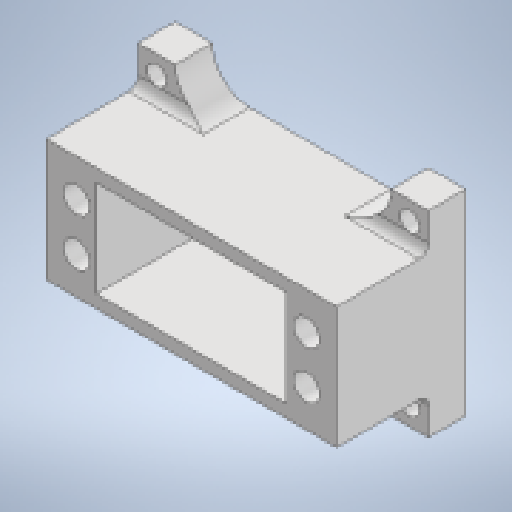
# Autodesk Inventor part: Soporte_Servo
Saved by Autodesk Inventor 2024 (Build 280153000, 153)
## iProperties
Created: 2024-07-18
Part Number: Soporte_Servo
Material: Genérico
Document SubType Name: Modelado
Designer: sergi
Density: 1 g/cm^3
Appearance: Valor por defecto
Sheet Metal Rule: Por defecto
Author: sergi
Autodesk Inventor part; units mm, degrees
ref_plane "YZ Plane" through (0, 0, 0) normal (1, 0, 0) x (0, 1, 0)
ref_plane "XZ Plane" through (0, 0, 0) normal (0, 1, 0) x (-1, 0, 0)
sketch "Boceto1" plane through (0, 0, 0) normal (0, 0, 1) x (1, 0, 0)
  line L0 (-20.0665, -74.268) -> (20.3335, -74.268) projected
  line L1 (-20.0665, -54.068) -> (-20.0665, -74.268) projected
  line L2 (20.3335, -74.268) -> (20.3335, -54.068) projected
  circle A0 centre (24.7835, -69.268) radius 2.2 projected
  circle A1 centre (24.7835, -59.068) radius 2.2 projected
  line L3 (20.3335, -54.068) -> (20.3335, -74.268) projected
  line L4 (20.3335, -54.068) -> (28.3335, -54.068) projected
  line L5 (28.3335, -54.068) -> (28.3335, -74.268) projected
  line L6 (20.3335, -74.268) -> (28.3335, -74.268) projected
  line L7 (-20.0665, -74.268) -> (-28.0665, -74.268) projected
  circle A2 centre (-24.5165, -69.268) radius 2.2 projected
  circle A3 centre (-24.5165, -59.068) radius 2.2 projected
  line L8 (-20.0665, -54.068) -> (-20.0665, -74.268) projected
  line L9 (-20.0665, -54.068) -> (-28.0665, -54.068) projected
  line L10 (-28.0665, -74.268) -> (-28.0665, -54.068) projected
  line L11 (-20.0665, -74.268) -> (-28.0665, -74.268) projected
  line L12 (-20.0665, -66.768) -> (-25.0665, -66.768) projected
  line L13 (-25.0665, -61.568) -> (-25.0665, -66.768) projected
  line L14 (-20.0665, -61.568) -> (-25.0665, -61.568) projected
  line L15 (-20.0665, -54.068) -> (-20.0665, -74.268) projected
  line L16 (20.3335, -54.068) -> (-20.0665, -54.068) projected
  line L17 (20.3335, -74.268) -> (20.3335, -54.068) projected
  line L18 (-20.0665, -74.268) -> (20.3335, -74.268) projected
  circle A4 centre (-10.3665, -64.168) radius 3.1 projected
  line L19 (-28.0665, -74.268) -> (-28.0665, -77.268)
  line L20 (-28.0665, -77.268) -> (-31.0665, -77.268)
  line L21 (28.3335, -54.068) -> (31.3335, -54.068)
  line L22 (31.3335, -54.068) -> (31.3335, -51.068)
  line L23 (31.3335, -51.068) -> (28.3335, -51.068)
  line L24 (28.3335, -51.068) -> (28.3335, -54.068)
  line L25 (31.3335, -51.068) -> (-31.0665, -51.068)
  line L26 (-31.0665, -51.068) -> (-31.0665, -77.268)
  line L27 (-31.0665, -77.268) -> (31.3335, -77.268)
  line L28 (31.3335, -77.268) -> (31.3335, -51.068)
  line L29 (-31.0665, -51.068) -> (-23.0665, -51.068)
  line L30 (-23.0665, -51.068) -> (-23.0665, -43.068)
  line L31 (-23.0665, -43.068) -> (-31.0665, -43.068)
  line L32 (-31.0665, -43.068) -> (-31.0665, -51.068)
  line L33 (-31.0665, -77.268) -> (-23.0665, -77.268)
  line L34 (-23.0665, -77.268) -> (-23.0665, -85.268)
  line L35 (-23.0665, -85.268) -> (-31.0665, -85.268)
  line L36 (-31.0665, -85.268) -> (-31.0665, -77.268)
  line L37 (31.3335, -77.268) -> (23.3335, -77.268)
  line L38 (23.3335, -77.268) -> (23.3335, -85.268)
  line L39 (23.3335, -85.268) -> (31.3335, -85.268)
  line L40 (31.3335, -85.268) -> (31.3335, -77.268)
  line L41 (31.3335, -51.068) -> (23.3335, -51.068)
  line L42 (23.3335, -51.068) -> (23.3335, -43.068)
  line L43 (23.3335, -43.068) -> (31.3335, -43.068)
  line L44 (31.3335, -43.068) -> (31.3335, -51.068)
  line L45 (-27.0665, -43.068) -> (-27.0665, -47.068)
  circle A5 centre (-27.0665, -47.068) radius 2.1
  line L46 (-27.0665, -85.268) -> (-27.0665, -81.268)
  circle A6 centre (-27.0665, -81.268) radius 2.1
  line L47 (27.3335, -43.068) -> (27.3335, -47.068)
  circle A7 centre (27.3335, -47.068) radius 2.1
  line L48 (27.3335, -85.268) -> (27.3335, -81.268)
  circle A8 centre (27.3335, -81.268) radius 2.1
  line L49 (-28.0665, -54.068) -> (28.3335, -54.068)
  line L50 (28.3335, -54.068) -> (28.3335, -74.268)
  line L51 (28.3335, -74.268) -> (-28.0665, -74.268)
  line L52 (-28.0665, -74.268) -> (-28.0665, -54.068)
  line L53 (28.5835, -53.818) -> (-28.3165, -53.818)
  line L54 (-28.3165, -53.818) -> (-28.3165, -74.518)
  line L55 (-28.3165, -74.518) -> (28.5835, -74.518)
  line L56 (28.5835, -74.518) -> (28.5835, -53.818)
  line L57 (-20.3165, -53.818) -> (-20.3165, -74.518)
  line L58 (20.5835, -74.518) -> (20.5835, -53.818)
  line L59 (-25.0665, -61.568) -> (-20.0665, -66.768)
  line L60 (-19.0665, -69.168) -> (-26.0665, -69.168)
  line L61 (-26.0665, -69.168) -> (-26.0665, -59.168)
  line L62 (-26.0665, -59.168) -> (-19.0665, -59.168)
  line L63 (-19.0665, -59.168) -> (-19.0665, -69.168)
  line L64 (-19.0665, -69.168) -> (-26.0665, -59.168) construction
  line L65 (-26.0665, -69.168) -> (-19.0665, -59.168) construction
  point P0 (0, 0)
  point P1 (28.5835, -54.068)
  point P2 (28.3335, -53.818)
  point P3 (-20.3165, -61.568)
  point P4 (-20.3165, -66.768)
  point P5 (-22.5665, -64.168)
  point P6 (-20.3165, -69.168)
  point P7 (-20.3165, -59.168)
  dimension "d0" = 3
  dimension "d1" = 3
  dimension "d2" = 3
  dimension "d3" = 3
  dimension "d4" = 8
  dimension "d5" = 8
  dimension "d6" = 8
  dimension "d7" = 8
  dimension "d8" = 8
  dimension "d9" = 8
  dimension "d10" = 8
  dimension "d11" = 8
  dimension "d12" = 4
  dimension "d13" = 4.2
  dimension "d14" = 4
  dimension "d15" = 4.2
  dimension "d16" = 4
  dimension "d17" = 4.2
  dimension "d18" = 4
  dimension "d19" = 4.2
  dimension "d20" = 0.25
  dimension "d28" = 0.25
  dimension "d29" = 0.25
  dimension "d30" = 7
  dimension "d31" = 10
  constraints: 94 end point, 20 parallel, 10 perpendicular, 8 horizontal, 5 midpoint, 5 vertical, 4 centre point, 4 coincident, 4 point on line, 3 other
  measures "d0" distance of L7.end L19.end
  measures "d1" distance of L19.end L20.end
  measures "d2" distance of L23.end L22.end
  measures "d3" distance of L22.end L21.end
  measures "d4" distance of L31.end L30.end
  measures "d5" distance of L30.end L29.end
  measures "d6" distance of L34.end L35.end
  measures "d7" distance of L33.end L34.end
  measures "d8" distance of L39.end L38.end
  measures "d9" distance of L38.end L37.end
  measures "d10" distance of L42.end L43.end
  measures "d11" distance of L41.end L42.end
  measures "d12" distance of L45.start L45.end
  measures "d13" diameter of A5
  measures "d14" distance of L46.start L46.end
  measures "d15" diameter of A6
  measures "d16" distance of L47.start L47.end
  measures "d17" diameter of A7
  measures "d18" distance of L48.start L48.end
  measures "d19" diameter of A8
  measures "d20" distance between parallel lines of L49 L53
  measures "d28" distance between parallel lines of L1 L57
  measures "d29" distance between parallel lines of L2 L58
  measures "d30" distance of L61.end L62.end
  measures "d31" distance of L60.end L61.end
extrude "Extrusión1" add sketch "Boceto1" along normal blind 8 contours L57 L55 L19 L7 | L7 L10 L9 L57 L62 A3 L61 A2 L60 | L58 L4 L5 L6 | L6 L5 L21 L56 L55 L58 | L19 L55 L54 L53 L57 L9 L10 | L55 L56 L21 L28 L27 L19 | L58 L53 L24 L4 | A2 L61 L60 | L19 L20 L26 L25 L24 L53 L54 L55 | L24 L53 L56 L21 | L27 L34 L35 L36 L20 | L56 L53 L24 L23 L22 L21 | A3 L62 L61 | L25 L42 L43 L44 L23 | L32 L31 L30 L25 | L27 L40 L39 L38 | A0 | A1 picked at (-23.5885, -69.413) picked at (-23.5885, -58.923)
sketch "Boceto2" plane through (0, 0, 8) normal (0, 0, 1) x (1, 0, 0)
  line L0 (-23.0665, -85.268) -> (-23.0665, -77.268) projected
  line L1 (-23.0665, -77.268) -> (23.3335, -77.268) projected
  line L2 (23.3335, -77.268) -> (23.3335, -85.268) projected
  line L3 (23.3335, -85.268) -> (31.3335, -85.268) projected
  line L4 (31.3335, -85.268) -> (31.3335, -43.068) projected
  line L5 (31.3335, -43.068) -> (23.3335, -43.068) projected
  line L6 (23.3335, -43.068) -> (23.3335, -51.068) projected
  line L7 (23.3335, -51.068) -> (-23.0665, -51.068) projected
  line L8 (-23.0665, -51.068) -> (-23.0665, -43.068) projected
  line L9 (-23.0665, -43.068) -> (-31.0665, -43.068) projected
  line L10 (-31.0665, -43.068) -> (-31.0665, -85.268) projected
  line L11 (-31.0665, -85.268) -> (-23.0665, -85.268) projected
  circle A0 centre (-27.0665, -81.268) radius 2.1 projected
  line L12 (20.5835, -74.518) -> (-20.3165, -74.518) projected
  line L13 (-20.3165, -53.818) -> (20.5835, -53.818) projected
  circle A1 centre (27.3335, -81.268) radius 2.1 projected
  circle A2 centre (-27.0665, -47.068) radius 2.1 projected
  circle A3 centre (27.3335, -47.068) radius 2.1 projected
  line L14 (-23.0665, -85.268) -> (-23.0665, -77.268) projected
  line L15 (-23.0665, -77.268) -> (-31.0665, -77.268)
  line L16 (-23.0665, -77.268) -> (-15.0665, -77.268) construction
  line L17 (23.3335, -51.068) -> (31.3335, -51.068)
  line L18 (31.3335, -85.268) -> (31.3335, -43.068) projected
  line L19 (23.3335, -51.068) -> (31.3335, -51.068) construction
  line L20 (-31.0665, -77.268) -> (31.3335, -77.268)
  line L21 (31.3335, -77.268) -> (31.3335, -51.068)
  line L22 (31.3335, -51.068) -> (-31.0665, -51.068)
  line L23 (-31.0665, -51.068) -> (-31.0665, -77.268)
  line L24 (20.5835, -53.818) -> (20.5835, -74.518) projected
  line L25 (-20.3165, -74.518) -> (-20.3165, -69.168) projected
  line L26 (-20.3165, -59.168) -> (-20.3165, -53.818) projected
  line L27 (-20.3165, -69.168) -> (-26.0665, -69.168) projected
  line L28 (-26.0665, -69.168) -> (-26.0665, -59.168) projected
  line L29 (-26.0665, -59.168) -> (-20.3165, -59.168) projected
  line L30 (-20.3165, -59.168) -> (-20.3165, -69.168)
  point P0 (0, 0)
  dimension "d23" = 180
  dimension "d24" = 8
  dimension "d25" = 0
  constraints: 18 end point, 3 horizontal, 2 collinear, 2 parallel, 2 perpendicular, 1 point on line, 1 vertical
  measures "d23" angle of L15 L16
  measures "d24" distance of L6.end L17.end
  measures "d25" distance between parallel lines of L17 L19
ref_plane "Plano de trabajo1" through (-28.0665, -74.268, 27.7) normal (0, 0, -1) x (0, 1, 0)
extrude "Extrusión2" add sketch "Boceto2" along normal up to surface (19.7 mm away) contours L15 L10 L22 L7 L17 L4 L20 L1 | L27 L28 L29 L30
sketch "Boceto3" plane through (-31.0665, -85.268, 0) normal (-1, 0, 0) x (0, 0, 1)
  line L0 (8, 16.1) -> (8, 26.1) projected
  line L1 (0, 26.1) -> (8, 26.1) projected
  line L2 (0, 26.1) -> (8, 26.1)
  line L3 (8, 26.1) -> (8, 16.1)
  line L4 (8, 16.1) -> (0, 16.1)
  line L5 (0, 16.1) -> (0, 26.1)
  point P0 (0, 85.268)
  constraints: 8 end point, 2 parallel, 1 horizontal, 1 perpendicular
extrude "Extrusión3" cut sketch "Boceto3" against normal blind 8
sketch "Boceto4" plane through (-31.0665, -51.068, 27.7) normal (0, 0, 1) x (1, 0, 0)
  circle A0 centre (6.55, -18.2) radius 2.2 projected
  circle A1 centre (6.55, -8) radius 2.2 projected
  line L0 (11, -3) -> (11, -23.2) projected
  line L1 (11, -3) -> (3, -3) projected
  line L2 (3, -23.2) -> (3, -3) projected
  line L3 (11, -23.2) -> (3, -23.2) projected
  circle A2 centre (55.85, -18.2) radius 2.2 projected
  circle A3 centre (55.85, -8) radius 2.2 projected
  line L4 (51.4, -23.2) -> (51.4, -3) projected
  line L5 (51.4, -23.2) -> (59.4, -23.2) projected
  line L6 (59.4, -23.2) -> (59.4, -3) projected
  line L7 (51.4, -3) -> (59.4, -3) projected
  point P0 (31.0665, 51.068)
hole "Agujero1" at (-24.5165, -69.268, 27.7) at (-24.5165, -59.068, 27.7) at (24.7835, -69.268, 27.7) at (24.7835, -59.068, 27.7) direction (0, 0, -1) diameter 5.6 depth 15
fillet "Empalme1" radius 8 4 edges at (-23.0665, -77.268, 4) (23.3335, -77.268, 4) (-23.0665, -51.068, 4) (23.3335, -51.068, 4)
fillet "Empalme2" radius 2 4 edges at (-19.0668, -77.268, 8) (19.3337, -77.268, 8) (19.3337, -51.068, 8) (-19.0668, -51.068, 8)
equation "\"Radio_pliegue\" = Grosor"
equation "\"Anchura_desahogo_plegado\" = Grosor"
equation "\"Profundidad_desahogo_plegado\" = 0.5 * Grosor"
equation "\"Tamaño_destalonado\" = 4 * Grosor"
equation "\"Remanente_mínimo\" = 2 * Grosor"
equation "\"Radiodetransición\" = Radio_pliegue"
equation "\"Tamaño_de_radio_de_Jacobi\" = Radio_pliegue"
equation "\"TamañoSeparación\" = Grosor"
equation "\"Grosor\" = 3.048"
